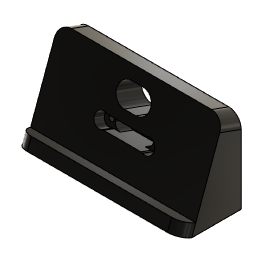
esp-module-ou (Autodesk Fusion 360 archive; units mm, degrees)
design "esp-module-ou-dock"
Autodesk Fusion 360 part; units mm, degrees
sketch "Sketch1" plane through (0, 0, 0) normal (0, 1, 0) x (1, 0, 0)
  line L0 (35, 0) -> (-35, 0)
  line L1 (-35, 0) -> (-35, -40)
  line L2 (-35, -40) -> (35, -40)
  line L3 (35, -40) -> (35, 0)
  line L4 (0, -40) -> (0, 0) construction
  line L5 (-11.1562, -16.2) -> (11.1562, -16.2)
  line L6 (11.1562, -16.2) -> (11.1562, -21.5) construction
  line L7 (11.1562, -21.5) -> (-11.1562, -21.5)
  line L8 (-11.1562, -21.5) -> (-11.1562, -16.2) construction
  line L9 (-5.35, -16.2) -> (-5.35, -21.5) construction
  line L10 (5.35, -16.2) -> (5.35, -21.5) construction
  line L11 (-11.1562, -18.85) -> (11.1562, -18.85) construction
  circle A0 centre (-9.75, -18.85) radius 3
  circle A1 centre (9.75, -18.85) radius 3
  line L12 (-8, -16.2) -> (-8, -21.5) construction
  line L13 (8, -16.2) -> (8, -21.5) construction
  circle A2 centre (-9.75, -18.85) radius 1
  arc A3 (-5.35, -16.2) -> (-5.35, -21.5) centre (-5.35, -18.85) ccw
  arc A4 (5.35, -21.5) -> (5.35, -16.2) centre (5.35, -18.85) ccw
  circle A5 centre (9.75, -18.85) radius 1
  line L14 (-35, -5) -> (35, -5)
  line L15 (-2.5, -35.15) -> (2.5, -35.15)
  line L16 (2.5, -35.15) -> (2.5, -25.65) construction
  line L17 (2.5, -25.65) -> (-2.5, -25.65)
  line L18 (-2.5, -25.65) -> (-2.5, -35.15) construction
  arc A6 (-2.5, -25.65) -> (-2.5, -35.15) centre (-2.5, -30.4) ccw
  arc A7 (2.5, -35.15) -> (2.5, -25.65) centre (2.5, -30.4) ccw
  line L19 (-7.25, -30.4) -> (7.25, -30.4) construction
  circle A8 centre (0, -18.85) radius 2
  dimension "d2" = 5.3
  dimension "d3" = 19.5
  dimension "d4" = 6
  dimension "d5" = 2
  dimension "d6" = 40
  dimension "d7" = 70
  dimension "d8" = 5
  dimension "d9" = 16
  dimension "d12" = 9.5
  dimension "d13" = 11.55
  dimension "d16" = 4
  dimension "d17" = 14.5
  dimension "d38" = 13.85
  constraint horizontal L0
  constraint vertical L1
  constraint horizontal L2
  constraint vertical L3
  constraint midpoint L2 L4.start
  constraint midpoint L0 L4.end
  constraint coincident L4.end origin
  constraint horizontal L5
  constraint vertical L6
  constraint horizontal L7
  constraint vertical L8
  constraint coincident L5 L9.start
  constraint coincident L7 L9.end
  constraint perpendicular L7 L9
  constraint coincident L5 L10.start
  constraint coincident L7 L10.end
  constraint perpendicular L7 L10
  constraint midpoint L8 L11.start
  constraint midpoint L6 L11.end
  constraint symmetric L4 L9 L10
  constraint coincident L11 A0.centre
  constraint coincident L5.start A0
  constraint coincident L11 A1.centre
  constraint coincident L5.end A1
  constraint symmetric L4 A0 A1
  constraint coincident L5 L12.start
  constraint coincident L7 L12.end
  constraint perpendicular L7 L12
  constraint coincident L5 L13.start
  constraint coincident L7 L13.end
  constraint perpendicular L7 L13
  constraint concentric A0 A2
  constraint midpoint L9 A3.centre
  constraint midpoint L10 A4.centre
  constraint concentric A1 A5
  constraint symmetric L4 A2 A5
  constraint coincident L1 L14.start
  constraint coincident L3 L14.end
  constraint perpendicular L3 L14
  constraint tangent L12 A3
  constraint tangent L13 A4
  constraint horizontal L15
  constraint vertical L16
  constraint horizontal L17
  constraint vertical L18
  constraint midpoint A6 L19.start
  constraint midpoint A7 L19.end
  constraint coincident L18 A6.centre
  constraint coincident L16 A7.centre
  constraint midpoint L11 A8.centre
  constraint symmetric L4 L16 L18
  measures "d2" distance of L5.start L7.end
  measures "d3" distance of A0.centre A1.centre
  measures "d4" diameter of A0
  measures "d5" diameter of A2
  measures "d6" distance of L0.end L1.end
  measures "d7" distance of L1.end L2.end
  measures "d8" distance of L0.end L14.start
  measures "d9" distance of L12.end L13.end
  measures "d12" distance of L15.start L17.end
  measures "d13" vertical distance of L11.end L19.end
  measures "d16" diameter of A8
  measures "d17" distance of L19.start L19.end
  measures "d38" distance of L11.end L14
extrude "Extrude1" add sketch "Sketch1" against normal blind 4.7 contours L0 L1 L3 L14 | L1 L2 L3 L14
extrude "Extrude2" add sketch "Sketch1" along normal blind 15 contours L0 L1 L3 L14 | L1 L2 L3 L14 | L5 A0 A3 | L5 L7 A0 A1 A3 A4 | L5 A1 A4 | L5 L7 A0 A3 | L5 A0 | A0 A3 | L5 A1 | L5 L7 A1 A4 | A1 A4 | L7 A0 A3 | L7 A1 A4 | L7 A0 | L7 A1 | A2 | A5
extrude "Extrude3" cut sketch "Sketch1" along normal blind 6 contours L5 L7 A0 A1 A3 A4 | A0 A3 | A1 A4
extrude "Extrude4" add sketch "Sketch1" against normal blind 10 contours L0 L1 L3 L14
extrude "Extrude5" cut sketch "Sketch1" along normal blind 5 contours A2 | A5
fillet "Fillet1" radius 2 4 edges at (-8.3438, -2.35, 21.5) (8.3438, -2.35, 21.5) (-8.3438, -2.35, 16.2) (8.3438, -2.35, 16.2)
fillet "Fillet3" radius 5.3 4 edges at (35, 5.15, 40) (-35, 5.15, 40) (-35, -10, 2.5) (35, -10, 2.5)
move_body "Move1" bodies 1 to x (1, 0, 0) y (0, 0.939693, -0.34202) z (0, 0.34202, 0.939693) at (0, -0.2834, -1.6075)
chamfer "Chamfer1" distance 7.17 angle 70 1 edges at (0, 13.8119, -6.7378) measured on face at (-25.5379, 20.963, 12.9096)
draft "Draft1" angle -20 neutral plane through (35, 5.7824, -0.0002) pull (0, 0, -1) 1 faces at (-25.6406, 21.8534, 15.3558)
equation "d2 = 4.8 mm + Shrinkage"
equation "d4 = 5.5 mm + Shrinkage"
equation "d5 = 1.5 mm + Shrinkage"
equation "d9 = 15.5 mm + Shrinkage"
equation "d12 = 9 mm + Shrinkage"
equation "d13 = 21.95 mm - Version"
equation "Shrinkage = 0.5 mm"
equation "Version = 10.4 mm"
equation "d17 = 14 mm + Shrinkage"
